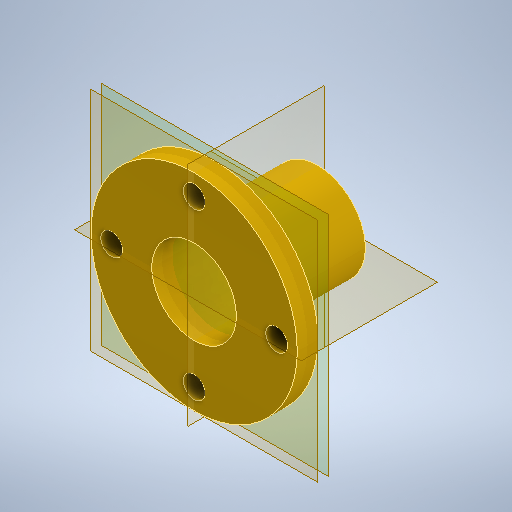
# Autodesk Inventor part: porca_roscada_trapezoidal_001
Saved by Autodesk Inventor 2026 (Build 300175000, 175)
## iProperties
Created: 2025-11-26
Part Number: porca_roscada_trapezoidal_001
Material: Aluminum 6061
Document SubType Name: Modeling
Designer: Carlos Dias
Density: 2.7 g/cm^3
Appearance: Gold
Author: Carlos Dias
Autodesk Inventor part; units mm, degrees
sketch "Sketch1" plane through (0, 0, 0) normal (0, 0, 1) x (1, 0, 0)
  circle A0 centre (0, 0) radius 4.1
  circle A1 centre (0, 0) radius 10
  circle A2 centre (0, 8) radius 1.05
  circle A3 centre (-8, 0) radius 1.05
  circle A4 centre (0, -8) radius 1.05
  circle A5 centre (8, 0) radius 1.05
  dimension "d0" = 8.2
  dimension "d7" = 20
  dimension "d33" = 2.1
  dimension "d34" = 8
  dimension "d37" = 360
  constraints: 6 centre point, 2 coincident, 1 vertical alignment, 9 other
  measures "d0" diameter of A0
  measures "d7" diameter of A1
  measures "d33" diameter of A2
  measures "d34" distance of point (0, 0) A2.centre
ref_plane "Work Plane5" through (0, 0, -1) normal (0, 0, -1) x (-1, 0, 0)
sketch "Sketch5" plane through (0, 0, -1) normal (0, 0, -1) x (-1, 0, 0)
  circle A0 centre (0, 0) radius 4.1 projected
  circle A1 centre (0, 0) radius 4.6
  dimension "d30" = 0.5
  constraints: 1 centre point
  measures "d30" radial gap between concentric circles of A0 A1
extrude "Extrusion8" add sketch "Sketch5" along normal blind 10
extrude "Extrusion9" add sketch "Sketch1" along normal mid plane 2
body "Solid3"
